Autodesk Inventor part; units mm, degrees
(part 2 of 4)
sketch "Sketch2" plane through (0, 0, 15) normal (0, 0, 1) x (1, 0, 0)
  line L0 (0, 0) -> (0, 2.4)
  line L1 (0, 2.4) -> (-192, 2.4)
  line L2 (-192, 2.4) -> (-192, 0)
  arc A0 (-192, 0) -> (-191.1122, 0.9525) centre (-192, 0.89) ccw
  arc A1 (-190.8628, 1.22) -> (-191.1122, 0.9525) centre (-190.8628, 0.97) ccw
  line L3 (-190.8628, 1.22) -> (-190.1372, 1.22)
  arc A2 (-189.8878, 0.9525) -> (-190.1372, 1.22) centre (-190.1372, 0.97) ccw
  arc A3 (-189.8878, 0.9525) -> (-188.1122, 0.9525) centre (-189, 0.89) ccw
  arc A4 (-187.8628, 1.22) -> (-188.1122, 0.9525) centre (-187.8628, 0.97) ccw
  line L4 (-187.8628, 1.22) -> (-187.1372, 1.22)
  arc A5 (-186.8878, 0.9525) -> (-187.1372, 1.22) centre (-187.1372, 0.97) ccw
  arc A6 (-186.8878, 0.9525) -> (-185.1122, 0.9525) centre (-186, 0.89) ccw
  arc A7 (-184.8628, 1.22) -> (-185.1122, 0.9525) centre (-184.8628, 0.97) ccw
  line L5 (-184.8628, 1.22) -> (-184.1372, 1.22)
  arc A8 (-183.8878, 0.9525) -> (-184.1372, 1.22) centre (-184.1372, 0.97) ccw
  arc A9 (-183.8878, 0.9525) -> (-182.1122, 0.9525) centre (-183, 0.89) ccw
  arc A10 (-181.8628, 1.22) -> (-182.1122, 0.9525) centre (-181.8628, 0.97) ccw
  line L6 (-181.8628, 1.22) -> (-181.1372, 1.22)
  arc A11 (-180.8878, 0.9525) -> (-181.1372, 1.22) centre (-181.1372, 0.97) ccw
  arc A12 (-180.8878, 0.9525) -> (-179.1122, 0.9525) centre (-180, 0.89) ccw
  arc A13 (-178.8628, 1.22) -> (-179.1122, 0.9525) centre (-178.8628, 0.97) ccw
  line L7 (-178.8628, 1.22) -> (-178.1372, 1.22)
  arc A14 (-177.8878, 0.9525) -> (-178.1372, 1.22) centre (-178.1372, 0.97) ccw
  arc A15 (-177.8878, 0.9525) -> (-176.1122, 0.9525) centre (-177, 0.89) ccw
  arc A16 (-175.8628, 1.22) -> (-176.1122, 0.9525) centre (-175.8628, 0.97) ccw
  line L8 (-175.8628, 1.22) -> (-175.1372, 1.22)
  arc A17 (-174.8878, 0.9525) -> (-175.1372, 1.22) centre (-175.1372, 0.97) ccw
  arc A18 (-174.8878, 0.9525) -> (-173.1122, 0.9525) centre (-174, 0.89) ccw
  arc A19 (-172.8628, 1.22) -> (-173.1122, 0.9525) centre (-172.8628, 0.97) ccw
  line L9 (-172.8628, 1.22) -> (-172.1372, 1.22)
  arc A20 (-171.8878, 0.9525) -> (-172.1372, 1.22) centre (-172.1372, 0.97) ccw
  arc A21 (-171.8878, 0.9525) -> (-170.1122, 0.9525) centre (-171, 0.89) ccw
  arc A22 (-169.8628, 1.22) -> (-170.1122, 0.9525) centre (-169.8628, 0.97) ccw
  line L10 (-169.8628, 1.22) -> (-169.1372, 1.22)
  arc A23 (-168.8878, 0.9525) -> (-169.1372, 1.22) centre (-169.1372, 0.97) ccw
  arc A24 (-168.8878, 0.9525) -> (-167.1122, 0.9525) centre (-168, 0.89) ccw
  arc A25 (-166.8628, 1.22) -> (-167.1122, 0.9525) centre (-166.8628, 0.97) ccw
  line L11 (-166.8628, 1.22) -> (-166.1372, 1.22)
  arc A26 (-165.8878, 0.9525) -> (-166.1372, 1.22) centre (-166.1372, 0.97) ccw
  arc A27 (-165.8878, 0.9525) -> (-164.1122, 0.9525) centre (-165, 0.89) ccw
  arc A28 (-163.8628, 1.22) -> (-164.1122, 0.9525) centre (-163.8628, 0.97) ccw
  line L12 (-163.8628, 1.22) -> (-163.1372, 1.22)
  arc A29 (-162.8878, 0.9525) -> (-163.1372, 1.22) centre (-163.1372, 0.97) ccw
  arc A30 (-162.8878, 0.9525) -> (-161.1122, 0.9525) centre (-162, 0.89) ccw
  arc A31 (-160.8628, 1.22) -> (-161.1122, 0.9525) centre (-160.8628, 0.97) ccw
  line L13 (-160.8628, 1.22) -> (-160.1372, 1.22)
  arc A32 (-159.8878, 0.9525) -> (-160.1372, 1.22) centre (-160.1372, 0.97) ccw
  arc A33 (-159.8878, 0.9525) -> (-158.1122, 0.9525) centre (-159, 0.89) ccw
  arc A34 (-157.8628, 1.22) -> (-158.1122, 0.9525) centre (-157.8628, 0.97) ccw
  line L14 (-157.8628, 1.22) -> (-157.1372, 1.22)
  arc A35 (-156.8878, 0.9525) -> (-157.1372, 1.22) centre (-157.1372, 0.97) ccw
  arc A36 (-156.8878, 0.9525) -> (-155.1122, 0.9525) centre (-156, 0.89) ccw
  arc A37 (-154.8628, 1.22) -> (-155.1122, 0.9525) centre (-154.8628, 0.97) ccw
  line L15 (-154.8628, 1.22) -> (-154.1372, 1.22)
  arc A38 (-153.8878, 0.9525) -> (-154.1372, 1.22) centre (-154.1372, 0.97) ccw
  arc A39 (-153.8878, 0.9525) -> (-152.1122, 0.9525) centre (-153, 0.89) ccw
  arc A40 (-151.8628, 1.22) -> (-152.1122, 0.9525) centre (-151.8628, 0.97) ccw
  line L16 (-151.8628, 1.22) -> (-151.1372, 1.22)
  arc A41 (-150.8878, 0.9525) -> (-151.1372, 1.22) centre (-151.1372, 0.97) ccw
  arc A42 (-150.8878, 0.9525) -> (-149.1122, 0.9525) centre (-150, 0.89) ccw
  arc A43 (-148.8628, 1.22) -> (-149.1122, 0.9525) centre (-148.8628, 0.97) ccw
  line L17 (-148.8628, 1.22) -> (-148.1372, 1.22)
  arc A44 (-147.8878, 0.9525) -> (-148.1372, 1.22) centre (-148.1372, 0.97) ccw
  arc A45 (-147.8878, 0.9525) -> (-146.1122, 0.9525) centre (-147, 0.89) ccw
  arc A46 (-145.8628, 1.22) -> (-146.1122, 0.9525) centre (-145.8628, 0.97) ccw
  line L18 (-145.8628, 1.22) -> (-145.1372, 1.22)
  arc A47 (-144.8878, 0.9525) -> (-145.1372, 1.22) centre (-145.1372, 0.97) ccw
  arc A48 (-144.8878, 0.9525) -> (-143.1122, 0.9525) centre (-144, 0.89) ccw
  arc A49 (-142.8628, 1.22) -> (-143.1122, 0.9525) centre (-142.8628, 0.97) ccw
  line L19 (-142.8628, 1.22) -> (-142.1372, 1.22)
  arc A50 (-141.8878, 0.9525) -> (-142.1372, 1.22) centre (-142.1372, 0.97) ccw
  arc A51 (-141.8878, 0.9525) -> (-140.1122, 0.9525) centre (-141, 0.89) ccw
  arc A52 (-139.8628, 1.22) -> (-140.1122, 0.9525) centre (-139.8628, 0.97) ccw
  line L20 (-139.8628, 1.22) -> (-139.1372, 1.22)
  arc A53 (-138.8878, 0.9525) -> (-139.1372, 1.22) centre (-139.1372, 0.97) ccw
  arc A54 (-138.8878, 0.9525) -> (-137.1122, 0.9525) centre (-138, 0.89) ccw
  arc A55 (-136.8628, 1.22) -> (-137.1122, 0.9525) centre (-136.8628, 0.97) ccw
  line L21 (-136.8628, 1.22) -> (-136.1372, 1.22)
  arc A56 (-135.8878, 0.9525) -> (-136.1372, 1.22) centre (-136.1372, 0.97) ccw
  arc A57 (-135.8878, 0.9525) -> (-134.1122, 0.9525) centre (-135, 0.89) ccw
  arc A58 (-133.8628, 1.22) -> (-134.1122, 0.9525) centre (-133.8628, 0.97) ccw
  line L22 (-133.8628, 1.22) -> (-133.1372, 1.22)
  arc A59 (-132.8878, 0.9525) -> (-133.1372, 1.22) centre (-133.1372, 0.97) ccw
  arc A60 (-132.8878, 0.9525) -> (-131.1122, 0.9525) centre (-132, 0.89) ccw
  arc A61 (-130.8628, 1.22) -> (-131.1122, 0.9525) centre (-130.8628, 0.97) ccw
  line L23 (-130.8628, 1.22) -> (-130.1372, 1.22)
  arc A62 (-129.8878, 0.9525) -> (-130.1372, 1.22) centre (-130.1372, 0.97) ccw
  arc A63 (-129.8878, 0.9525) -> (-128.1122, 0.9525) centre (-129, 0.89) ccw
  arc A64 (-127.8628, 1.22) -> (-128.1122, 0.9525) centre (-127.8628, 0.97) ccw
  line L24 (-127.8628, 1.22) -> (-127.1372, 1.22)
  arc A65 (-126.8878, 0.9525) -> (-127.1372, 1.22) centre (-127.1372, 0.97) ccw
  arc A66 (-126.8878, 0.9525) -> (-125.1122, 0.9525) centre (-126, 0.89) ccw
  arc A67 (-124.8628, 1.22) -> (-125.1122, 0.9525) centre (-124.8628, 0.97) ccw
  line L25 (-124.8628, 1.22) -> (-124.1372, 1.22)
  arc A68 (-123.8878, 0.9525) -> (-124.1372, 1.22) centre (-124.1372, 0.97) ccw
  arc A69 (-123.8878, 0.9525) -> (-122.1122, 0.9525) centre (-123, 0.89) ccw
  arc A70 (-121.8628, 1.22) -> (-122.1122, 0.9525) centre (-121.8628, 0.97) ccw
  line L26 (-121.8628, 1.22) -> (-121.1372, 1.22)
  arc A71 (-120.8878, 0.9525) -> (-121.1372, 1.22) centre (-121.1372, 0.97) ccw
  arc A72 (-120.8878, 0.9525) -> (-119.1122, 0.9525) centre (-120, 0.89) ccw
  arc A73 (-118.8628, 1.22) -> (-119.1122, 0.9525) centre (-118.8628, 0.97) ccw
  line L27 (-118.8628, 1.22) -> (-118.1372, 1.22)
  arc A74 (-117.8878, 0.9525) -> (-118.1372, 1.22) centre (-118.1372, 0.97) ccw
  arc A75 (-117.8878, 0.9525) -> (-116.1122, 0.9525) centre (-117, 0.89) ccw
  arc A76 (-115.8628, 1.22) -> (-116.1122, 0.9525) centre (-115.8628, 0.97) ccw
  line L28 (-115.8628, 1.22) -> (-115.1372, 1.22)
  arc A77 (-114.8878, 0.9525) -> (-115.1372, 1.22) centre (-115.1372, 0.97) ccw
  arc A78 (-114.8878, 0.9525) -> (-113.1122, 0.9525) centre (-114, 0.89) ccw
  arc A79 (-112.8628, 1.22) -> (-113.1122, 0.9525) centre (-112.8628, 0.97) ccw
  line L29 (-112.8628, 1.22) -> (-112.1372, 1.22)
  arc A80 (-111.8878, 0.9525) -> (-112.1372, 1.22) centre (-112.1372, 0.97) ccw
  arc A81 (-111.8878, 0.9525) -> (-110.1122, 0.9525) centre (-111, 0.89) ccw
  arc A82 (-109.8628, 1.22) -> (-110.1122, 0.9525) centre (-109.8628, 0.97) ccw
  line L30 (-109.8628, 1.22) -> (-109.1372, 1.22)
  arc A83 (-108.8878, 0.9525) -> (-109.1372, 1.22) centre (-109.1372, 0.97) ccw
  arc A84 (-108.8878, 0.9525) -> (-107.1122, 0.9525) centre (-108, 0.89) ccw
  arc A85 (-106.8628, 1.22) -> (-107.1122, 0.9525) centre (-106.8628, 0.97) ccw
  line L31 (-106.8628, 1.22) -> (-106.1372, 1.22)
  arc A86 (-105.8878, 0.9525) -> (-106.1372, 1.22) centre (-106.1372, 0.97) ccw
  arc A87 (-105.8878, 0.9525) -> (-104.1122, 0.9525) centre (-105, 0.89) ccw
  arc A88 (-103.8628, 1.22) -> (-104.1122, 0.9525) centre (-103.8628, 0.97) ccw
  line L32 (-103.8628, 1.22) -> (-103.1372, 1.22)
  arc A89 (-102.8878, 0.9525) -> (-103.1372, 1.22) centre (-103.1372, 0.97) ccw
  arc A90 (-102.8878, 0.9525) -> (-101.1122, 0.9525) centre (-102, 0.89) ccw
  arc A91 (-100.8628, 1.22) -> (-101.1122, 0.9525) centre (-100.8628, 0.97) ccw
  line L33 (-100.8628, 1.22) -> (-100.1372, 1.22)
  arc A92 (-99.8878, 0.9525) -> (-100.1372, 1.22) centre (-100.1372, 0.97) ccw
  arc A93 (-99.8878, 0.9525) -> (-98.1122, 0.9525) centre (-99, 0.89) ccw
  arc A94 (-97.8628, 1.22) -> (-98.1122, 0.9525) centre (-97.8628, 0.97) ccw
  line L34 (-97.8628, 1.22) -> (-97.1372, 1.22)
  arc A95 (-96.8878, 0.9525) -> (-97.1372, 1.22) centre (-97.1372, 0.97) ccw
  arc A96 (-96.8878, 0.9525) -> (-95.1122, 0.9525) centre (-96, 0.89) ccw
  arc A97 (-94.8628, 1.22) -> (-95.1122, 0.9525) centre (-94.8628, 0.97) ccw
  line L35 (-94.8628, 1.22) -> (-94.1372, 1.22)
  arc A98 (-93.8878, 0.9525) -> (-94.1372, 1.22) centre (-94.1372, 0.97) ccw
  arc A99 (-93.8878, 0.9525) -> (-92.1122, 0.9525) centre (-93, 0.89) ccw
  arc A100 (-91.8628, 1.22) -> (-92.1122, 0.9525) centre (-91.8628, 0.97) ccw
  line L36 (-91.8628, 1.22) -> (-91.1372, 1.22)
  arc A101 (-90.8878, 0.9525) -> (-91.1372, 1.22) centre (-91.1372, 0.97) ccw
  arc A102 (-90.8878, 0.9525) -> (-89.1122, 0.9525) centre (-90, 0.89) ccw
  arc A103 (-88.8628, 1.22) -> (-89.1122, 0.9525) centre (-88.8628, 0.97) ccw
  line L37 (-88.8628, 1.22) -> (-88.1372, 1.22)
  arc A104 (-87.8878, 0.9525) -> (-88.1372, 1.22) centre (-88.1372, 0.97) ccw
  arc A105 (-87.8878, 0.9525) -> (-86.1122, 0.9525) centre (-87, 0.89) ccw
  arc A106 (-85.8628, 1.22) -> (-86.1122, 0.9525) centre (-85.8628, 0.97) ccw
  line L38 (-85.8628, 1.22) -> (-85.1372, 1.22)
  arc A107 (-84.8878, 0.9525) -> (-85.1372, 1.22) centre (-85.1372, 0.97) ccw
  arc A108 (-84.8878, 0.9525) -> (-83.1122, 0.9525) centre (-84, 0.89) ccw
  arc A109 (-82.8628, 1.22) -> (-83.1122, 0.9525) centre (-82.8628, 0.97) ccw
  line L39 (-82.8628, 1.22) -> (-82.1372, 1.22)
  arc A110 (-81.8878, 0.9525) -> (-82.1372, 1.22) centre (-82.1372, 0.97) ccw
  arc A111 (-81.8878, 0.9525) -> (-80.1122, 0.9525) centre (-81, 0.89) ccw
  arc A112 (-79.8628, 1.22) -> (-80.1122, 0.9525) centre (-79.8628, 0.97) ccw
  line L40 (-79.8628, 1.22) -> (-79.1372, 1.22)
  arc A113 (-78.8878, 0.9525) -> (-79.1372, 1.22) centre (-79.1372, 0.97) ccw
  arc A114 (-78.8878, 0.9525) -> (-77.1122, 0.9525) centre (-78, 0.89) ccw
  arc A115 (-76.8628, 1.22) -> (-77.1122, 0.9525) centre (-76.8628, 0.97) ccw
  line L41 (-76.8628, 1.22) -> (-76.1372, 1.22)
  arc A116 (-75.8878, 0.9525) -> (-76.1372, 1.22) centre (-76.1372, 0.97) ccw
  arc A117 (-75.8878, 0.9525) -> (-74.1122, 0.9525) centre (-75, 0.89) ccw
  arc A118 (-73.8628, 1.22) -> (-74.1122, 0.9525) centre (-73.8628, 0.97) ccw
  line L42 (-73.8628, 1.22) -> (-73.1372, 1.22)
  arc A119 (-72.8878, 0.9525) -> (-73.1372, 1.22) centre (-73.1372, 0.97) ccw
  arc A120 (-72.8878, 0.9525) -> (-71.1122, 0.9525) centre (-72, 0.89) ccw
  arc A121 (-70.8628, 1.22) -> (-71.1122, 0.9525) centre (-70.8628, 0.97) ccw
  line L43 (-70.8628, 1.22) -> (-70.1372, 1.22)
  arc A122 (-69.8878, 0.9525) -> (-70.1372, 1.22) centre (-70.1372, 0.97) ccw
  arc A123 (-69.8878, 0.9525) -> (-68.1122, 0.9525) centre (-69, 0.89) ccw
  arc A124 (-67.8628, 1.22) -> (-68.1122, 0.9525) centre (-67.8628, 0.97) ccw
  line L44 (-67.8628, 1.22) -> (-67.1372, 1.22)
  arc A125 (-66.8878, 0.9525) -> (-67.1372, 1.22) centre (-67.1372, 0.97) ccw
  arc A126 (-66.8878, 0.9525) -> (-65.1122, 0.9525) centre (-66, 0.89) ccw
  arc A127 (-64.8628, 1.22) -> (-65.1122, 0.9525) centre (-64.8628, 0.97) ccw
  line L45 (-64.8628, 1.22) -> (-64.1372, 1.22)
  arc A128 (-63.8878, 0.9525) -> (-64.1372, 1.22) centre (-64.1372, 0.97) ccw
  arc A129 (-63.8878, 0.9525) -> (-62.1122, 0.9525) centre (-63, 0.89) ccw
  arc A130 (-61.8628, 1.22) -> (-62.1122, 0.9525) centre (-61.8628, 0.97) ccw
  line L46 (-61.8628, 1.22) -> (-61.1372, 1.22)
  arc A131 (-60.8878, 0.9525) -> (-61.1372, 1.22) centre (-61.1372, 0.97) ccw
  arc A132 (-60.8878, 0.9525) -> (-59.1122, 0.9525) centre (-60, 0.89) ccw
  arc A133 (-58.8628, 1.22) -> (-59.1122, 0.9525) centre (-58.8628, 0.97) ccw
  line L47 (-58.8628, 1.22) -> (-58.1372, 1.22)
  arc A134 (-57.8878, 0.9525) -> (-58.1372, 1.22) centre (-58.1372, 0.97) ccw
  arc A135 (-57.8878, 0.9525) -> (-56.1122, 0.9525) centre (-57, 0.89) ccw
  arc A136 (-55.8628, 1.22) -> (-56.1122, 0.9525) centre (-55.8628, 0.97) ccw
  line L48 (-55.8628, 1.22) -> (-55.1372, 1.22)
  arc A137 (-54.8878, 0.9525) -> (-55.1372, 1.22) centre (-55.1372, 0.97) ccw
  arc A138 (-54.8878, 0.9525) -> (-53.1122, 0.9525) centre (-54, 0.89) ccw
  arc A139 (-52.8628, 1.22) -> (-53.1122, 0.9525) centre (-52.8628, 0.97) ccw
  line L49 (-52.8628, 1.22) -> (-52.1372, 1.22)
  arc A140 (-51.8878, 0.9525) -> (-52.1372, 1.22) centre (-52.1372, 0.97) ccw
  arc A141 (-51.8878, 0.9525) -> (-50.1122, 0.9525) centre (-51, 0.89) ccw
  arc A142 (-49.8628, 1.22) -> (-50.1122, 0.9525) centre (-49.8628, 0.97) ccw
  line L50 (-49.8628, 1.22) -> (-49.1372, 1.22)
  arc A143 (-48.8878, 0.9525) -> (-49.1372, 1.22) centre (-49.1372, 0.97) ccw
  arc A144 (-48.8878, 0.9525) -> (-47.1122, 0.9525) centre (-48, 0.89) ccw
  arc A145 (-46.8628, 1.22) -> (-47.1122, 0.9525) centre (-46.8628, 0.97) ccw
  line L51 (-46.8628, 1.22) -> (-46.1372, 1.22)
  arc A146 (-45.8878, 0.9525) -> (-46.1372, 1.22) centre (-46.1372, 0.97) ccw
  arc A147 (-45.8878, 0.9525) -> (-44.1122, 0.9525) centre (-45, 0.89) ccw
  arc A148 (-43.8628, 1.22) -> (-44.1122, 0.9525) centre (-43.8628, 0.97) ccw
  line L52 (-43.8628, 1.22) -> (-43.1372, 1.22)
  arc A149 (-42.8878, 0.9525) -> (-43.1372, 1.22) centre (-43.1372, 0.97) ccw
  arc A150 (-42.8878, 0.9525) -> (-41.1122, 0.9525) centre (-42, 0.89) ccw
  arc A151 (-40.8628, 1.22) -> (-41.1122, 0.9525) centre (-40.8628, 0.97) ccw
  line L53 (-40.8628, 1.22) -> (-40.1372, 1.22)
  arc A152 (-39.8878, 0.9525) -> (-40.1372, 1.22) centre (-40.1372, 0.97) ccw
  arc A153 (-39.8878, 0.9525) -> (-38.1122, 0.9525) centre (-39, 0.89) ccw
  arc A154 (-37.8628, 1.22) -> (-38.1122, 0.9525) centre (-37.8628, 0.97) ccw
  line L54 (-37.8628, 1.22) -> (-37.1372, 1.22)
  arc A155 (-36.8878, 0.9525) -> (-37.1372, 1.22) centre (-37.1372, 0.97) ccw
  arc A156 (-36.8878, 0.9525) -> (-35.1122, 0.9525) centre (-36, 0.89) ccw
  arc A157 (-34.8628, 1.22) -> (-35.1122, 0.9525) centre (-34.8628, 0.97) ccw
  line L55 (-34.8628, 1.22) -> (-34.1372, 1.22)
  arc A158 (-33.8878, 0.9525) -> (-34.1372, 1.22) centre (-34.1372, 0.97) ccw
  arc A159 (-33.8878, 0.9525) -> (-32.1122, 0.9525) centre (-33, 0.89) ccw
  arc A160 (-31.8628, 1.22) -> (-32.1122, 0.9525) centre (-31.8628, 0.97) ccw
  line L56 (-31.8628, 1.22) -> (-31.1372, 1.22)
  arc A161 (-30.8878, 0.9525) -> (-31.1372, 1.22) centre (-31.1372, 0.97) ccw
  arc A162 (-30.8878, 0.9525) -> (-29.1122, 0.9525) centre (-30, 0.89) ccw
  arc A163 (-28.8628, 1.22) -> (-29.1122, 0.9525) centre (-28.8628, 0.97) ccw
  line L57 (-28.8628, 1.22) -> (-28.1372, 1.22)
  arc A164 (-27.8878, 0.9525) -> (-28.1372, 1.22) centre (-28.1372, 0.97) ccw
  arc A165 (-27.8878, 0.9525) -> (-26.1122, 0.9525) centre (-27, 0.89) ccw
  arc A166 (-25.8628, 1.22) -> (-26.1122, 0.9525) centre (-25.8628, 0.97) ccw
  line L58 (-25.8628, 1.22) -> (-25.1372, 1.22)
  arc A167 (-24.8878, 0.9525) -> (-25.1372, 1.22) centre (-25.1372, 0.97) ccw
  arc A168 (-24.8878, 0.9525) -> (-23.1122, 0.9525) centre (-24, 0.89) ccw
  arc A169 (-22.8628, 1.22) -> (-23.1122, 0.9525) centre (-22.8628, 0.97) ccw
  line L59 (-22.8628, 1.22) -> (-22.1372, 1.22)
  arc A170 (-21.8878, 0.9525) -> (-22.1372, 1.22) centre (-22.1372, 0.97) ccw
  arc A171 (-21.8878, 0.9525) -> (-20.1122, 0.9525) centre (-21, 0.89) ccw
  arc A172 (-19.8628, 1.22) -> (-20.1122, 0.9525) centre (-19.8628, 0.97) ccw
  line L60 (-19.8628, 1.22) -> (-19.1372, 1.22)
  arc A173 (-18.8878, 0.9525) -> (-19.1372, 1.22) centre (-19.1372, 0.97) ccw
  arc A174 (-18.8878, 0.9525) -> (-17.1122, 0.9525) centre (-18, 0.89) ccw
  arc A175 (-16.8628, 1.22) -> (-17.1122, 0.9525) centre (-16.8628, 0.97) ccw
  line L61 (-16.8628, 1.22) -> (-16.1372, 1.22)
  arc A176 (-15.8878, 0.9525) -> (-16.1372, 1.22) centre (-16.1372, 0.97) ccw
  arc A177 (-15.8878, 0.9525) -> (-14.1122, 0.9525) centre (-15, 0.89) ccw
  arc A178 (-13.8628, 1.22) -> (-14.1122, 0.9525) centre (-13.8628, 0.97) ccw
  line L62 (-13.8628, 1.22) -> (-13.1372, 1.22)
  arc A179 (-12.8878, 0.9525) -> (-13.1372, 1.22) centre (-13.1372, 0.97) ccw
  arc A180 (-12.8878, 0.9525) -> (-11.1122, 0.9525) centre (-12, 0.89) ccw
  arc A181 (-10.8628, 1.22) -> (-11.1122, 0.9525) centre (-10.8628, 0.97) ccw
  line L63 (-10.8628, 1.22) -> (-10.1372, 1.22)
  arc A182 (-9.8878, 0.9525) -> (-10.1372, 1.22) centre (-10.1372, 0.97) ccw
  arc A183 (-9.8878, 0.9525) -> (-8.1122, 0.9525) centre (-9, 0.89) ccw
  arc A184 (-7.8628, 1.22) -> (-8.1122, 0.9525) centre (-7.8628, 0.97) ccw
  line L64 (-7.8628, 1.22) -> (-7.1372, 1.22)
  arc A185 (-6.8878, 0.9525) -> (-7.1372, 1.22) centre (-7.1372, 0.97) ccw
  arc A186 (-6.8878, 0.9525) -> (-5.1122, 0.9525) centre (-6, 0.89) ccw
  arc A187 (-4.8628, 1.22) -> (-5.1122, 0.9525) centre (-4.8628, 0.97) ccw
  line L65 (-4.8628, 1.22) -> (-4.1372, 1.22)
  arc A188 (-3.8878, 0.9525) -> (-4.1372, 1.22) centre (-4.1372, 0.97) ccw
  arc A189 (-3.8878, 0.9525) -> (-2.1122, 0.9525) centre (-3, 0.89) ccw
  arc A190 (-1.8628, 1.22) -> (-2.1122, 0.9525) centre (-1.8628, 0.97) ccw
  line L66 (-1.8628, 1.22) -> (-1.1372, 1.22)
  arc A191 (-0.8878, 0.9525) -> (-1.1372, 1.22) centre (-1.1372, 0.97) ccw
  arc A192 (-0.8878, 0.9525) -> (0, 0) centre (0, 0.89) ccw
  line L67 (-384, 0) -> (-384, 2.4)
  line L68 (-384, 2.4) -> (-192, 2.4)
  arc A193 (-192.8878, 0.9525) -> (-192, 0) centre (-192, 0.89) ccw
  arc A194 (-192.8878, 0.9525) -> (-193.1372, 1.22) centre (-193.1372, 0.97) ccw
  line L69 (-193.1372, 1.22) -> (-193.8628, 1.22)
  arc A195 (-193.8628, 1.22) -> (-194.1122, 0.9525) centre (-193.8628, 0.97) ccw
  arc A196 (-195.8878, 0.9525) -> (-194.1122, 0.9525) centre (-195, 0.89) ccw
  arc A197 (-195.8878, 0.9525) -> (-196.1372, 1.22) centre (-196.1372, 0.97) ccw
  line L70 (-196.1372, 1.22) -> (-196.8628, 1.22)
  arc A198 (-196.8628, 1.22) -> (-197.1122, 0.9525) centre (-196.8628, 0.97) ccw
  arc A199 (-198.8878, 0.9525) -> (-197.1122, 0.9525) centre (-198, 0.89) ccw
  arc A200 (-198.8878, 0.9525) -> (-199.1372, 1.22) centre (-199.1372, 0.97) ccw
  line L71 (-199.1372, 1.22) -> (-199.8628, 1.22)
  arc A201 (-199.8628, 1.22) -> (-200.1122, 0.9525) centre (-199.8628, 0.97) ccw
  arc A202 (-201.8878, 0.9525) -> (-200.1122, 0.9525) centre (-201, 0.89) ccw
  arc A203 (-201.8878, 0.9525) -> (-202.1372, 1.22) centre (-202.1372, 0.97) ccw
  line L72 (-202.1372, 1.22) -> (-202.8628, 1.22)
  arc A204 (-202.8628, 1.22) -> (-203.1122, 0.9525) centre (-202.8628, 0.97) ccw
  arc A205 (-204.8878, 0.9525) -> (-203.1122, 0.9525) centre (-204, 0.89) ccw
  arc A206 (-204.8878, 0.9525) -> (-205.1372, 1.22) centre (-205.1372, 0.97) ccw
  line L73 (-205.1372, 1.22) -> (-205.8628, 1.22)
  arc A207 (-205.8628, 1.22) -> (-206.1122, 0.9525) centre (-205.8628, 0.97) ccw
  arc A208 (-207.8878, 0.9525) -> (-206.1122, 0.9525) centre (-207, 0.89) ccw
  arc A209 (-207.8878, 0.9525) -> (-208.1372, 1.22) centre (-208.1372, 0.97) ccw
  line L74 (-208.1372, 1.22) -> (-208.8628, 1.22)
  arc A210 (-208.8628, 1.22) -> (-209.1122, 0.9525) centre (-208.8628, 0.97) ccw
  arc A211 (-210.8878, 0.9525) -> (-209.1122, 0.9525) centre (-210, 0.89) ccw
  arc A212 (-210.8878, 0.9525) -> (-211.1372, 1.22) centre (-211.1372, 0.97) ccw
  line L75 (-211.1372, 1.22) -> (-211.8628, 1.22)
  arc A213 (-211.8628, 1.22) -> (-212.1122, 0.9525) centre (-211.8628, 0.97) ccw
  arc A214 (-213.8878, 0.9525) -> (-212.1122, 0.9525) centre (-213, 0.89) ccw
  arc A215 (-213.8878, 0.9525) -> (-214.1372, 1.22) centre (-214.1372, 0.97) ccw
  line L76 (-214.1372, 1.22) -> (-214.8628, 1.22)
  arc A216 (-214.8628, 1.22) -> (-215.1122, 0.9525) centre (-214.8628, 0.97) ccw
  arc A217 (-216.8878, 0.9525) -> (-215.1122, 0.9525) centre (-216, 0.89) ccw
  arc A218 (-216.8878, 0.9525) -> (-217.1372, 1.22) centre (-217.1372, 0.97) ccw
  line L77 (-217.1372, 1.22) -> (-217.8628, 1.22)
  arc A219 (-217.8628, 1.22) -> (-218.1122, 0.9525) centre (-217.8628, 0.97) ccw
  arc A220 (-219.8878, 0.9525) -> (-218.1122, 0.9525) centre (-219, 0.89) ccw
  arc A221 (-219.8878, 0.9525) -> (-220.1372, 1.22) centre (-220.1372, 0.97) ccw
  line L78 (-220.1372, 1.22) -> (-220.8628, 1.22)
  arc A222 (-220.8628, 1.22) -> (-221.1122, 0.9525) centre (-220.8628, 0.97) ccw
  arc A223 (-222.8878, 0.9525) -> (-221.1122, 0.9525) centre (-222, 0.89) ccw
  arc A224 (-222.8878, 0.9525) -> (-223.1372, 1.22) centre (-223.1372, 0.97) ccw
  line L79 (-223.1372, 1.22) -> (-223.8628, 1.22)
  arc A225 (-223.8628, 1.22) -> (-224.1122, 0.9525) centre (-223.8628, 0.97) ccw
  arc A226 (-225.8878, 0.9525) -> (-224.1122, 0.9525) centre (-225, 0.89) ccw
  arc A227 (-225.8878, 0.9525) -> (-226.1372, 1.22) centre (-226.1372, 0.97) ccw
  line L80 (-226.1372, 1.22) -> (-226.8628, 1.22)
  arc A228 (-226.8628, 1.22) -> (-227.1122, 0.9525) centre (-226.8628, 0.97) ccw
  arc A229 (-228.8878, 0.9525) -> (-227.1122, 0.9525) centre (-228, 0.89) ccw
  arc A230 (-228.8878, 0.9525) -> (-229.1372, 1.22) centre (-229.1372, 0.97) ccw
  line L81 (-229.1372, 1.22) -> (-229.8628, 1.22)
  arc A231 (-229.8628, 1.22) -> (-230.1122, 0.9525) centre (-229.8628, 0.97) ccw
  arc A232 (-231.8878, 0.9525) -> (-230.1122, 0.9525) centre (-231, 0.89) ccw
  arc A233 (-231.8878, 0.9525) -> (-232.1372, 1.22) centre (-232.1372, 0.97) ccw
  line L82 (-232.1372, 1.22) -> (-232.8628, 1.22)
  arc A234 (-232.8628, 1.22) -> (-233.1122, 0.9525) centre (-232.8628, 0.97) ccw
  arc A235 (-234.8878, 0.9525) -> (-233.1122, 0.9525) centre (-234, 0.89) ccw
  arc A236 (-234.8878, 0.9525) -> (-235.1372, 1.22) centre (-235.1372, 0.97) ccw
  line L83 (-235.1372, 1.22) -> (-235.8628, 1.22)
  arc A237 (-235.8628, 1.22) -> (-236.1122, 0.9525) centre (-235.8628, 0.97) ccw
  arc A238 (-237.8878, 0.9525) -> (-236.1122, 0.9525) centre (-237, 0.89) ccw
  arc A239 (-237.8878, 0.9525) -> (-238.1372, 1.22) centre (-238.1372, 0.97) ccw
  line L84 (-238.1372, 1.22) -> (-238.8628, 1.22)
  arc A240 (-238.8628, 1.22) -> (-239.1122, 0.9525) centre (-238.8628, 0.97) ccw
  arc A241 (-240.8878, 0.9525) -> (-239.1122, 0.9525) centre (-240, 0.89) ccw
  arc A242 (-240.8878, 0.9525) -> (-241.1372, 1.22) centre (-241.1372, 0.97) ccw
  line L85 (-241.1372, 1.22) -> (-241.8628, 1.22)
  arc A243 (-241.8628, 1.22) -> (-242.1122, 0.9525) centre (-241.8628, 0.97) ccw
  arc A244 (-243.8878, 0.9525) -> (-242.1122, 0.9525) centre (-243, 0.89) ccw
  arc A245 (-243.8878, 0.9525) -> (-244.1372, 1.22) centre (-244.1372, 0.97) ccw
  line L86 (-244.1372, 1.22) -> (-244.8628, 1.22)
  arc A246 (-244.8628, 1.22) -> (-245.1122, 0.9525) centre (-244.8628, 0.97) ccw
  arc A247 (-246.8878, 0.9525) -> (-245.1122, 0.9525) centre (-246, 0.89) ccw
  arc A248 (-246.8878, 0.9525) -> (-247.1372, 1.22) centre (-247.1372, 0.97) ccw
  line L87 (-247.1372, 1.22) -> (-247.8628, 1.22)
  arc A249 (-247.8628, 1.22) -> (-248.1122, 0.9525) centre (-247.8628, 0.97) ccw
  arc A250 (-249.8878, 0.9525) -> (-248.1122, 0.9525) centre (-249, 0.89) ccw
  arc A251 (-249.8878, 0.9525) -> (-250.1372, 1.22) centre (-250.1372, 0.97) ccw
  line L88 (-250.1372, 1.22) -> (-250.8628, 1.22)
  arc A252 (-250.8628, 1.22) -> (-251.1122, 0.9525) centre (-250.8628, 0.97) ccw
  arc A253 (-252.8878, 0.9525) -> (-251.1122, 0.9525) centre (-252, 0.89) ccw
  arc A254 (-252.8878, 0.9525) -> (-253.1372, 1.22) centre (-253.1372, 0.97) ccw
  line L89 (-253.1372, 1.22) -> (-253.8628, 1.22)
  arc A255 (-253.8628, 1.22) -> (-254.1122, 0.9525) centre (-253.8628, 0.97) ccw
  arc A256 (-255.8878, 0.9525) -> (-254.1122, 0.9525) centre (-255, 0.89) ccw
  arc A257 (-255.8878, 0.9525) -> (-256.1372, 1.22) centre (-256.1372, 0.97) ccw
  line L90 (-256.1372, 1.22) -> (-256.8628, 1.22)
  arc A258 (-256.8628, 1.22) -> (-257.1122, 0.9525) centre (-256.8628, 0.97) ccw
  arc A259 (-258.8878, 0.9525) -> (-257.1122, 0.9525) centre (-258, 0.89) ccw
  arc A260 (-258.8878, 0.9525) -> (-259.1372, 1.22) centre (-259.1372, 0.97) ccw
  line L91 (-259.1372, 1.22) -> (-259.8628, 1.22)
  arc A261 (-259.8628, 1.22) -> (-260.1122, 0.9525) centre (-259.8628, 0.97) ccw
  arc A262 (-261.8878, 0.9525) -> (-260.1122, 0.9525) centre (-261, 0.89) ccw
  arc A263 (-261.8878, 0.9525) -> (-262.1372, 1.22) centre (-262.1372, 0.97) ccw
  line L92 (-262.1372, 1.22) -> (-262.8628, 1.22)
  arc A264 (-262.8628, 1.22) -> (-263.1122, 0.9525) centre (-262.8628, 0.97) ccw
  arc A265 (-264.8878, 0.9525) -> (-263.1122, 0.9525) centre (-264, 0.89) ccw
  arc A266 (-264.8878, 0.9525) -> (-265.1372, 1.22) centre (-265.1372, 0.97) ccw
  line L93 (-265.1372, 1.22) -> (-265.8628, 1.22)
  arc A267 (-265.8628, 1.22) -> (-266.1122, 0.9525) centre (-265.8628, 0.97) ccw
  arc A268 (-267.8878, 0.9525) -> (-266.1122, 0.9525) centre (-267, 0.89) ccw
  arc A269 (-267.8878, 0.9525) -> (-268.1372, 1.22) centre (-268.1372, 0.97) ccw
  line L94 (-268.1372, 1.22) -> (-268.8628, 1.22)
  arc A270 (-268.8628, 1.22) -> (-269.1122, 0.9525) centre (-268.8628, 0.97) ccw
  arc A271 (-270.8878, 0.9525) -> (-269.1122, 0.9525) centre (-270, 0.89) ccw
  arc A272 (-270.8878, 0.9525) -> (-271.1372, 1.22) centre (-271.1372, 0.97) ccw
  line L95 (-271.1372, 1.22) -> (-271.8628, 1.22)
  arc A273 (-271.8628, 1.22) -> (-272.1122, 0.9525) centre (-271.8628, 0.97) ccw
  arc A274 (-273.8878, 0.9525) -> (-272.1122, 0.9525) centre (-273, 0.89) ccw
  arc A275 (-273.8878, 0.9525) -> (-274.1372, 1.22) centre (-274.1372, 0.97) ccw
  line L96 (-274.1372, 1.22) -> (-274.8628, 1.22)
  arc A276 (-274.8628, 1.22) -> (-275.1122, 0.9525) centre (-274.8628, 0.97) ccw
  arc A277 (-276.8878, 0.9525) -> (-275.1122, 0.9525) centre (-276, 0.89) ccw
  arc A278 (-276.8878, 0.9525) -> (-277.1372, 1.22) centre (-277.1372, 0.97) ccw
  line L97 (-277.1372, 1.22) -> (-277.8628, 1.22)
  arc A279 (-277.8628, 1.22) -> (-278.1122, 0.9525) centre (-277.8628, 0.97) ccw
  arc A280 (-279.8878, 0.9525) -> (-278.1122, 0.9525) centre (-279, 0.89) ccw
  arc A281 (-279.8878, 0.9525) -> (-280.1372, 1.22) centre (-280.1372, 0.97) ccw
  line L98 (-280.1372, 1.22) -> (-280.8628, 1.22)
  arc A282 (-280.8628, 1.22) -> (-281.1122, 0.9525) centre (-280.8628, 0.97) ccw
  arc A283 (-282.8878, 0.9525) -> (-281.1122, 0.9525) centre (-282, 0.89) ccw
  arc A284 (-282.8878, 0.9525) -> (-283.1372, 1.22) centre (-283.1372, 0.97) ccw
  line L99 (-283.1372, 1.22) -> (-283.8628, 1.22)
  arc A285 (-283.8628, 1.22) -> (-284.1122, 0.9525) centre (-283.8628, 0.97) ccw
  arc A286 (-285.8878, 0.9525) -> (-284.1122, 0.9525) centre (-285, 0.89) ccw
  arc A287 (-285.8878, 0.9525) -> (-286.1372, 1.22) centre (-286.1372, 0.97) ccw
  line L100 (-286.1372, 1.22) -> (-286.8628, 1.22)
  arc A288 (-286.8628, 1.22) -> (-287.1122, 0.9525) centre (-286.8628, 0.97) ccw
  arc A289 (-288.8878, 0.9525) -> (-287.1122, 0.9525) centre (-288, 0.89) ccw
  arc A290 (-288.8878, 0.9525) -> (-289.1372, 1.22) centre (-289.1372, 0.97) ccw
  line L101 (-289.1372, 1.22) -> (-289.8628, 1.22)
  arc A291 (-289.8628, 1.22) -> (-290.1122, 0.9525) centre (-289.8628, 0.97) ccw
  arc A292 (-291.8878, 0.9525) -> (-290.1122, 0.9525) centre (-291, 0.89) ccw
  arc A293 (-291.8878, 0.9525) -> (-292.1372, 1.22) centre (-292.1372, 0.97) ccw
  line L102 (-292.1372, 1.22) -> (-292.8628, 1.22)
  arc A294 (-292.8628, 1.22) -> (-293.1122, 0.9525) centre (-292.8628, 0.97) ccw
  arc A295 (-294.8878, 0.9525) -> (-293.1122, 0.9525) centre (-294, 0.89) ccw
  arc A296 (-294.8878, 0.9525) -> (-295.1372, 1.22) centre (-295.1372, 0.97) ccw
  line L103 (-295.1372, 1.22) -> (-295.8628, 1.22)
  arc A297 (-295.8628, 1.22) -> (-296.1122, 0.9525) centre (-295.8628, 0.97) ccw
  arc A298 (-297.8878, 0.9525) -> (-296.1122, 0.9525) centre (-297, 0.89) ccw
  arc A299 (-297.8878, 0.9525) -> (-298.1372, 1.22) centre (-298.1372, 0.97) ccw
  line L104 (-298.1372, 1.22) -> (-298.8628, 1.22)
  arc A300 (-298.8628, 1.22) -> (-299.1122, 0.9525) centre (-298.8628, 0.97) ccw
  arc A301 (-300.8878, 0.9525) -> (-299.1122, 0.9525) centre (-300, 0.89) ccw
  arc A302 (-300.8878, 0.9525) -> (-301.1372, 1.22) centre (-301.1372, 0.97) ccw
  line L105 (-301.1372, 1.22) -> (-301.8628, 1.22)
  arc A303 (-301.8628, 1.22) -> (-302.1122, 0.9525) centre (-301.8628, 0.97) ccw
  arc A304 (-303.8878, 0.9525) -> (-302.1122, 0.9525) centre (-303, 0.89) ccw
  arc A305 (-303.8878, 0.9525) -> (-304.1372, 1.22) centre (-304.1372, 0.97) ccw
  line L106 (-304.1372, 1.22) -> (-304.8628, 1.22)
  arc A306 (-304.8628, 1.22) -> (-305.1122, 0.9525) centre (-304.8628, 0.97) ccw
  arc A307 (-306.8878, 0.9525) -> (-305.1122, 0.9525) centre (-306, 0.89) ccw
  arc A308 (-306.8878, 0.9525) -> (-307.1372, 1.22) centre (-307.1372, 0.97) ccw
  line L107 (-307.1372, 1.22) -> (-307.8628, 1.22)
  arc A309 (-307.8628, 1.22) -> (-308.1122, 0.9525) centre (-307.8628, 0.97) ccw
  arc A310 (-309.8878, 0.9525) -> (-308.1122, 0.9525) centre (-309, 0.89) ccw
  arc A311 (-309.8878, 0.9525) -> (-310.1372, 1.22) centre (-310.1372, 0.97) ccw
  line L108 (-310.1372, 1.22) -> (-310.8628, 1.22)
  arc A312 (-310.8628, 1.22) -> (-311.1122, 0.9525) centre (-310.8628, 0.97) ccw
  arc A313 (-312.8878, 0.9525) -> (-311.1122, 0.9525) centre (-312, 0.89) ccw
  arc A314 (-312.8878, 0.9525) -> (-313.1372, 1.22) centre (-313.1372, 0.97) ccw
  line L109 (-313.1372, 1.22) -> (-313.8628, 1.22)
  arc A315 (-313.8628, 1.22) -> (-314.1122, 0.9525) centre (-313.8628, 0.97) ccw
  arc A316 (-315.8878, 0.9525) -> (-314.1122, 0.9525) centre (-315, 0.89) ccw
  arc A317 (-315.8878, 0.9525) -> (-316.1372, 1.22) centre (-316.1372, 0.97) ccw
  line L110 (-316.1372, 1.22) -> (-316.8628, 1.22)
  arc A318 (-316.8628, 1.22) -> (-317.1122, 0.9525) centre (-316.8628, 0.97) ccw
  arc A319 (-318.8878, 0.9525) -> (-317.1122, 0.9525) centre (-318, 0.89) ccw
  arc A320 (-318.8878, 0.9525) -> (-319.1372, 1.22) centre (-319.1372, 0.97) ccw
  line L111 (-319.1372, 1.22) -> (-319.8628, 1.22)
  arc A321 (-319.8628, 1.22) -> (-320.1122, 0.9525) centre (-319.8628, 0.97) ccw
  arc A322 (-321.8878, 0.9525) -> (-320.1122, 0.9525) centre (-321, 0.89) ccw
  arc A323 (-321.8878, 0.9525) -> (-322.1372, 1.22) centre (-322.1372, 0.97) ccw
  line L112 (-322.1372, 1.22) -> (-322.8628, 1.22)
  arc A324 (-322.8628, 1.22) -> (-323.1122, 0.9525) centre (-322.8628, 0.97) ccw
  arc A325 (-324.8878, 0.9525) -> (-323.1122, 0.9525) centre (-324, 0.89) ccw
  arc A326 (-324.8878, 0.9525) -> (-325.1372, 1.22) centre (-325.1372, 0.97) ccw
  line L113 (-325.1372, 1.22) -> (-325.8628, 1.22)
  arc A327 (-325.8628, 1.22) -> (-326.1122, 0.9525) centre (-325.8628, 0.97) ccw
  arc A328 (-327.8878, 0.9525) -> (-326.1122, 0.9525) centre (-327, 0.89) ccw
  arc A329 (-327.8878, 0.9525) -> (-328.1372, 1.22) centre (-328.1372, 0.97) ccw
  line L114 (-328.1372, 1.22) -> (-328.8628, 1.22)
  arc A330 (-328.8628, 1.22) -> (-329.1122, 0.9525) centre (-328.8628, 0.97) ccw
  arc A331 (-330.8878, 0.9525) -> (-329.1122, 0.9525) centre (-330, 0.89) ccw
  arc A332 (-330.8878, 0.9525) -> (-331.1372, 1.22) centre (-331.1372, 0.97) ccw
  line L115 (-331.1372, 1.22) -> (-331.8628, 1.22)
  arc A333 (-331.8628, 1.22) -> (-332.1122, 0.9525) centre (-331.8628, 0.97) ccw
  arc A334 (-333.8878, 0.9525) -> (-332.1122, 0.9525) centre (-333, 0.89) ccw
  arc A335 (-333.8878, 0.9525) -> (-334.1372, 1.22) centre (-334.1372, 0.97) ccw
  line L116 (-334.1372, 1.22) -> (-334.8628, 1.22)
  arc A336 (-334.8628, 1.22) -> (-335.1122, 0.9525) centre (-334.8628, 0.97) ccw
  arc A337 (-336.8878, 0.9525) -> (-335.1122, 0.9525) centre (-336, 0.89) ccw
  arc A338 (-336.8878, 0.9525) -> (-337.1372, 1.22) centre (-337.1372, 0.97) ccw
  line L117 (-337.1372, 1.22) -> (-337.8628, 1.22)
  arc A339 (-337.8628, 1.22) -> (-338.1122, 0.9525) centre (-337.8628, 0.97) ccw
  arc A340 (-339.8878, 0.9525) -> (-338.1122, 0.9525) centre (-339, 0.89) ccw
  arc A341 (-339.8878, 0.9525) -> (-340.1372, 1.22) centre (-340.1372, 0.97) ccw
  line L118 (-340.1372, 1.22) -> (-340.8628, 1.22)
  arc A342 (-340.8628, 1.22) -> (-341.1122, 0.9525) centre (-340.8628, 0.97) ccw
  arc A343 (-342.8878, 0.9525) -> (-341.1122, 0.9525) centre (-342, 0.89) ccw
  arc A344 (-342.8878, 0.9525) -> (-343.1372, 1.22) centre (-343.1372, 0.97) ccw
  line L119 (-343.1372, 1.22) -> (-343.8628, 1.22)
  arc A345 (-343.8628, 1.22) -> (-344.1122, 0.9525) centre (-343.8628, 0.97) ccw
  arc A346 (-345.8878, 0.9525) -> (-344.1122, 0.9525) centre (-345, 0.89) ccw
  arc A347 (-345.8878, 0.9525) -> (-346.1372, 1.22) centre (-346.1372, 0.97) ccw
  line L120 (-346.1372, 1.22) -> (-346.8628, 1.22)
  arc A348 (-346.8628, 1.22) -> (-347.1122, 0.9525) centre (-346.8628, 0.97) ccw
  arc A349 (-348.8878, 0.9525) -> (-347.1122, 0.9525) centre (-348, 0.89) ccw
  arc A350 (-348.8878, 0.9525) -> (-349.1372, 1.22) centre (-349.1372, 0.97) ccw
  line L121 (-349.1372, 1.22) -> (-349.8628, 1.22)
  arc A351 (-349.8628, 1.22) -> (-350.1122, 0.9525) centre (-349.8628, 0.97) ccw
  arc A352 (-351.8878, 0.9525) -> (-350.1122, 0.9525) centre (-351, 0.89) ccw
  arc A353 (-351.8878, 0.9525) -> (-352.1372, 1.22) centre (-352.1372, 0.97) ccw
  line L122 (-352.1372, 1.22) -> (-352.8628, 1.22)
  arc A354 (-352.8628, 1.22) -> (-353.1122, 0.9525) centre (-352.8628, 0.97) ccw
  arc A355 (-354.8878, 0.9525) -> (-353.1122, 0.9525) centre (-354, 0.89) ccw
  arc A356 (-354.8878, 0.9525) -> (-355.1372, 1.22) centre (-355.1372, 0.97) ccw
  line L123 (-355.1372, 1.22) -> (-355.8628, 1.22)
  arc A357 (-355.8628, 1.22) -> (-356.1122, 0.9525) centre (-355.8628, 0.97) ccw
  arc A358 (-357.8878, 0.9525) -> (-356.1122, 0.9525) centre (-357, 0.89) ccw
  arc A359 (-357.8878, 0.9525) -> (-358.1372, 1.22) centre (-358.1372, 0.97) ccw
  line L124 (-358.1372, 1.22) -> (-358.8628, 1.22)
  arc A360 (-358.8628, 1.22) -> (-359.1122, 0.9525) centre (-358.8628, 0.97) ccw
  arc A361 (-360.8878, 0.9525) -> (-359.1122, 0.9525) centre (-360, 0.89) ccw
  arc A362 (-360.8878, 0.9525) -> (-361.1372, 1.22) centre (-361.1372, 0.97) ccw
  line L125 (-361.1372, 1.22) -> (-361.8628, 1.22)
  arc A363 (-361.8628, 1.22) -> (-362.1122, 0.9525) centre (-361.8628, 0.97) ccw
  arc A364 (-363.8878, 0.9525) -> (-362.1122, 0.9525) centre (-363, 0.89) ccw
  arc A365 (-363.8878, 0.9525) -> (-364.1372, 1.22) centre (-364.1372, 0.97) ccw
  line L126 (-364.1372, 1.22) -> (-364.8628, 1.22)
  arc A366 (-364.8628, 1.22) -> (-365.1122, 0.9525) centre (-364.8628, 0.97) ccw
  arc A367 (-366.8878, 0.9525) -> (-365.1122, 0.9525) centre (-366, 0.89) ccw
  arc A368 (-366.8878, 0.9525) -> (-367.1372, 1.22) centre (-367.1372, 0.97) ccw
  line L127 (-367.1372, 1.22) -> (-367.8628, 1.22)
  arc A369 (-367.8628, 1.22) -> (-368.1122, 0.9525) centre (-367.8628, 0.97) ccw
  arc A370 (-369.8878, 0.9525) -> (-368.1122, 0.9525) centre (-369, 0.89) ccw
  arc A371 (-369.8878, 0.9525) -> (-370.1372, 1.22) centre (-370.1372, 0.97) ccw
  line L128 (-370.1372, 1.22) -> (-370.8628, 1.22)
  arc A372 (-370.8628, 1.22) -> (-371.1122, 0.9525) centre (-370.8628, 0.97) ccw
  arc A373 (-372.8878, 0.9525) -> (-371.1122, 0.9525) centre (-372, 0.89) ccw
  arc A374 (-372.8878, 0.9525) -> (-373.1372, 1.22) centre (-373.1372, 0.97) ccw
  line L129 (-373.1372, 1.22) -> (-373.8628, 1.22)
  arc A375 (-373.8628, 1.22) -> (-374.1122, 0.9525) centre (-373.8628, 0.97) ccw
  arc A376 (-375.8878, 0.9525) -> (-374.1122, 0.9525) centre (-375, 0.89) ccw
  arc A377 (-375.8878, 0.9525) -> (-376.1372, 1.22) centre (-376.1372, 0.97) ccw
  line L130 (-376.1372, 1.22) -> (-376.8628, 1.22)
  arc A378 (-376.8628, 1.22) -> (-377.1122, 0.9525) centre (-376.8628, 0.97) ccw
  arc A379 (-378.8878, 0.9525) -> (-377.1122, 0.9525) centre (-378, 0.89) ccw
  arc A380 (-378.8878, 0.9525) -> (-379.1372, 1.22) centre (-379.1372, 0.97) ccw
  line L131 (-379.1372, 1.22) -> (-379.8628, 1.22)
  arc A381 (-379.8628, 1.22) -> (-380.1122, 0.9525) centre (-379.8628, 0.97) ccw
  arc A382 (-381.8878, 0.9525) -> (-380.1122, 0.9525) centre (-381, 0.89) ccw
  arc A383 (-381.8878, 0.9525) -> (-382.1372, 1.22) centre (-382.1372, 0.97) ccw
  line L132 (-382.1372, 1.22) -> (-382.8628, 1.22)
  arc A384 (-382.8628, 1.22) -> (-383.1122, 0.9525) centre (-382.8628, 0.97) ccw
  arc A385 (-384, 0) -> (-383.1122, 0.9525) centre (-384, 0.89) ccw
  point P0 (0, 0)
  constraints: 451 symmetric about line, 386 point on circle, 193 centre point, 132 end point, 193 other
extrude "Extrusion2" add sketch "Sketch2" against normal blind 15 contours L2 A193 A194 L69 A195 A196 A197 L70 A198 A199 A200 L71 A201 A202 A203 L72 A204 A205 A206 L73 A207 A208 A209 L74 A210 A211 A212 L75 A213 A214 A215 L76 A216 A217 A218 L77 A219 A220 A221 L78 A222 A223 A224 L79 A225 A226 A227 L80 A228 A229 A230 L81 A231 A232 A233 L82 A234 A235 A236 L83 A237 A238 A239 L84 A240 A241 A242 L85 A243 A244 A245 L86 A246 A247 A248 L87 A249 A250 A251 L88 A252 A253 A254 L89 A255 A256 A257 L90 A258 A259 A260 L91 A261 A262 A263 L92 A264 A265 A266 L93 A267 A268 A269 L94 A270 A271 A272 L95 A273 A274 A275 L96 A276 A277 A278 L97 A279 A280 A281 L98 A282 A283 A284 L99 A285 A286 A287 L100 A288 A289 A290 L101 A291 A292 A293 L102 A294 A295 A296 L103 A297 A298 A299 L104 A300 A301 A302 L105 A303 A304 A305 L106 A306 A307 A308 L107 A309 A310 A311 L108 A312 A313 A314 L109 A315 A316 A317 L110 A318 A319 A320 L111 A321 A322 A323 L112 A324 A325 A326 L113 A327 A328 A329 L114 A330 A331 A332 L115 A333 A334 A335 L116 A336 A337 A338 L117 A339 A340 A341 L118 A342 A343 A344 L119 A345 A346 A347 L120 A348 A349 A350 L121 A351 A352 A353 L122 A354 A355 A356 L123 A357 A358 A359 L124 A360 A361 A362 L125 A363 A364 A365 L126 A366 A367 A368 L127 A369 A370 A371 L128 A372 A373 A374 L129 A375 A376 A377 L130 A378 A379 A380 L131 A381 A382 A383 L132 A384 A385 L67 L68